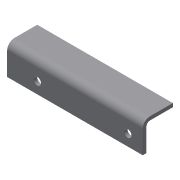
# Autodesk Inventor part: Chain Tension - L Bracket
Saved by Autodesk Inventor 2015 (Build 190159000, 159)
## iProperties
Created: 2015-02-01
Part Number: Chain Tension - L Bracket
Material: Generic
Document SubType Name: Sheet Metal
Designer: Tanner
Density: 1 g/cm^3
Sheet Metal Rule: Default
Appearance: Default
Author: Tanner
Autodesk Inventor part; units mm, degrees
ref_plane "YZ Plane" through (0, 0, 0) normal (1, 0, 0) x (0, 1, 0)
ref_plane "XZ Plane" through (0, 0, 0) normal (0, 1, 0) x (-1, 0, 0)
ref_plane "XY Plane" through (0, 0, 0) normal (0, 0, 1) x (1, 0, 0)
sketch "Sketch1" plane through (0, 0, 0) normal (0, 0, 1) x (1, 0, 0)
  line L0 (0, 0) -> (114.3, 0)
  line L1 (114.3, 0) -> (114.3, 25.4)
  line L2 (114.3, 25.4) -> (0, 25.4)
  line L3 (0, 25.4) -> (0, 0)
  dimension "d0" = 114.3
  dimension "d1" = 25.4
  measures "d0" distance of L2.end L1.end
  measures "d1" distance of L1.end L0.end
extrude "Plate1" add sketch "Sketch1" along normal blind 3.048
sketch "Sketch2" plane through (114.3, 22.352, 3.048) normal (0, 1, 0) x (-1, 0, 0)
  line L0 (114.3, 0) -> (0, 0)
  line L1 (0, 0) -> (0, -25.4)
  line L2 (0, -25.4) -> (114.3, -25.4)
  line L3 (114.3, -25.4) -> (114.3, 0)
  constraints: 6 end point, 1 horizontal, 1 perpendicular, 1 vertical
edge flange "Flange1" height 25.4 angle 90 thickness 3.048 bend radius 3.048 thickness toward (0, 1, 0) relief tear relief width 3.048 relief depth 1.524 edges at (57.15, 25.4, 0) wall of the first edge with corners at (0, 22.352, 3.048) (114.3, 22.352, 3.048) (114.3, 22.352, -22.352) (0, 22.352, -22.352)
bend "Bend1"
corner "Corner1"
hole "Hole1" at (101.6, 9.652, 0) direction (0, 0, 1) diameter 6.35 end through all
hole "Hole2" at (25.4, 9.652, 0) direction (0, 0, 1) diameter 6.35 end through all
equation "\"d20\" = Thickness"
equation "\"d29\" = Thickness"
equation "\"d3\" = BendReliefWidth"
equation "\"d4\" = BendReliefDepth"
equation "\"d5\" = MinimumRemnant"
equation "\"d6\" = BendRadius"
equation "\"d9\" = BendRadius"
equation "\"d10\" = CornerReliefSize"
equation "\"d11\" = GapSize"
equation "\"d12\" = JacobiRadiusSize"
equation "\"BendRadius\" = Thickness"
equation "\"BendReliefWidth\" = Thickness"
equation "\"BendReliefDepth\" = 0.5 * Thickness"
equation "\"CornerReliefSize\" = 4 * Thickness"
equation "\"MinimumRemnant\" = 2 * Thickness"
equation "\"TransitionRadius\" = BendRadius"
equation "\"JacobiRadiusSize\" = BendRadius"
equation "\"GapSize\" = Thickness"
equation "\"d2\" = BendRadius"
equation "\"Thickness\" = 3.048"
body "Solid1"
